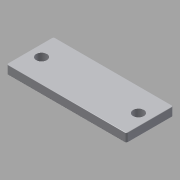
# Autodesk Inventor part: CIM Mount Top
Saved by Autodesk Inventor 2013 (Build 170138000, 138)
## iProperties
Created: 2013-01-18
Part Number: CIM Mount Top
Material: Aluminum 6061
Document SubType Name: Modeling
Designer: Naphat
Density: 1 g/cm^3
Author: Naphat
Autodesk Inventor part; units mm, degrees
ref_plane "YZ Plane" through (0, 0, 0) normal (1, 0, 0) x (0, 1, 0)
ref_plane "XZ Plane" through (0, 0, 0) normal (0, 1, 0) x (-1, 0, 0)
ref_plane "XY Plane" through (0, 0, 0) normal (0, 0, 1) x (1, 0, 0)
sketch "Sketch1" plane through (0, 0, 0) normal (0, 1, 0) x (-1, 0, 0)
  line L0 (0, 0) -> (284.48, 0)
  line L1 (284.48, 0) -> (284.48, 111.76)
  line L2 (284.48, 111.76) -> (0, 111.76)
  line L3 (0, 111.76) -> (0, 0)
  dimension "d0" = 284.48
  dimension "d1" = 111.76
  constraints: 8 end point, 2 perpendicular, 1 horizontal, 1 parallel
  measures "d0" distance of L0.start L0.end
  measures "d1" distance of L0.end L1.end
extrude "Extrusion1" add sketch "Sketch1" along normal blind 20.32
sketch "Sketch2" plane through (0, 20.32, 0) normal (0, 1, 0) x (1, 0, 0)
  line L0 (-284.48, 0) -> (-284.48, -111.76) projected
  line L1 (0, -111.76) -> (0, 0) projected
  line L2 (-284.48, -55.88) -> (-257.175, -55.88) construction
  line L3 (0, -55.88) -> (-27.305, -55.88) construction
  circle A0 centre (-27.305, -55.88) radius 12.7
  circle A1 centre (-257.175, -55.88) radius 12.7
  dimension "d4" = 27.305
  dimension "d5" = 27.305
  dimension "d6" = 25.4
  dimension "d7" = 25.4
  constraints: 4 end point, 2 centre point, 2 coincident, 2 midpoint, 1 collinear, 1 perpendicular
  measures "d4" distance of L2.start L2.end
  measures "d5" distance of L3.start L3.end
  measures "d6" diameter of A0
  measures "d7" diameter of A1
extrude "Extrusion2" cut sketch "Sketch2" against normal blind 20.32
fillet "Fillet1" radius 4 4 edges at (-284.48, 10.16, 111.76) (-284.48, 10.16, 0) (0, 10.16, 111.76) (0, 10.16, 0)
fillet "Fillet2" radius 1 16 edges at (-283.3084, 0, 1.1716) (-284.48, 0, 55.88) (-283.3084, 0, 110.5884) (-142.24, 0, 111.76) (-1.1716, 0, 110.5884) (0, 0, 55.88) (-1.1716, 0, 1.1716) (-142.24, 0, 0) (-283.3084, 20.32, 1.1716) (-284.48, 20.32, 55.88) (-283.3084, 20.32, 110.5884) (-142.24, 20.32, 111.76) (-1.1716, 20.32, 110.5884) (0, 20.32, 55.88) (-1.1716, 20.32, 1.1716) (-142.24, 20.32, 0)
equation "\"d5\" = d4"
body "Solid1"
